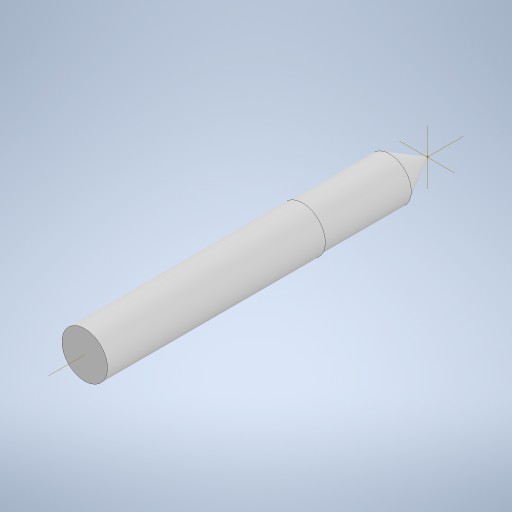
# Autodesk Inventor part: CPTCone
Saved by Autodesk Inventor 2023.1 (Build 271208000, 208)
## iProperties
Created: 2023-01-19
Part Number: CPTCone
Material: Generisch
Document SubType Name: Modeling
Designer: mehan
Density: 1 g/cm^3
Appearance: Vorgabe
Author: mehan
Autodesk Inventor part; units mm, degrees
ref_plane "YZ Plane" through (0, 0, 0) normal (1, 0, 0) x (0, 1, 0)
ref_plane "XZ Plane" through (0, 0, 0) normal (0, 1, 0) x (-1, 0, 0)
ref_plane "XY Plane" through (0, 0, 0) normal (0, 0, 1) x (1, 0, 0)
sketch "Skizze1" plane through (0, 0, 0) normal (1, 0, 0) x (0, 1, 0)
  line L0 (0, 0) -> (17.8, 0) construction
  line L1 (0, 0) -> (17.8, 30.8305)
  line L2 (0, 0) -> (35.6, 0) construction
  line L3 (17.8, 30.8305) -> (17.8, 66.4305)
  line L4 (17.8, 66.4305) -> (17.8, 102.0305)
  line L5 (18.69, 102.0305) -> (18.69, 280.0305)
  line L6 (18.69, 280.0305) -> (0, 280.0305)
  line L7 (17.8, 102.0305) -> (18.69, 102.0305)
  line L8 (0, 280.0305) -> (0, 0)
  dimension "d2" = 17.8
  dimension "d3" = 60
  dimension "d4" = 35.6
  dimension "d5" = 35.6
  dimension "d7" = 178
  constraints: 18 end point, 3 horizontal, 2 vertical, 1 equal length, 1 perpendicular, 1 point on line
  measures "d2" distance of L0.start L0.end
  measures "d3" angle of L2 L1
  measures "d4" distance of L1.end L3.end
  measures "d5" distance of L3.end L4.end
  measures "d7" distance of L5.start L5.end
revolve "Umdrehung1" add sketch "Skizze1" angle 360 about axis through (0, 0, 280.0305) along (0, 0, -1)
